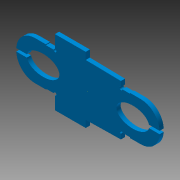
# Autodesk Inventor part: LockZ
Saved by Autodesk Inventor 2014 SP2 (Build 180246200, 246)
## iProperties
Created: 2014-11-24
Part Number: LockZ
Material: Generic
Document SubType Name: Modeling
Designer: JLM
Density: 1 g/cm^3
Appearance: Default
Author: JLM
Autodesk Inventor part; units mm, degrees
ref_plane "YZ Plane" through (0, 0, 0) normal (1, 0, 0) x (0, 1, 0)
ref_plane "XZ Plane" through (0, 0, 0) normal (0, 1, 0) x (-1, 0, 0)
ref_plane "XY Plane" through (0, 0, 0) normal (0, 0, 1) x (1, 0, 0)
sketch "Sketch1" plane through (0, 0, 0) normal (0, 0, 1) x (1, 0, 0)
  line L0 (48.35, 0) -> (48.35, 13.2)
  line L1 (48.35, 13.2) -> (28.35, 13.2)
  line L2 (28.35, 13.2) -> (28.35, 12.7)
  line L3 (28.35, 12.7) -> (22.25, 12.7)
  line L4 (12.2521, 0) -> (48.35, 0)
  line L5 (22.25, 12.7) -> (22.25, 22.25)
  line L6 (22.25, 22.25) -> (0, 22.25)
  line L7 (48.35, 1) -> (41.2045, 1)
  line L8 (48.35, 0) -> (48.35, -13.2)
  line L9 (48.35, -13.2) -> (28.35, -13.2)
  line L10 (28.35, -13.2) -> (28.35, -12.7)
  line L11 (28.35, -12.7) -> (22.25, -12.7)
  line L12 (22.25, -12.7) -> (22.25, -22.25)
  line L13 (22.25, -22.25) -> (0, -22.25)
  line L14 (48.35, -1) -> (41.2045, -1)
  line L15 (0, 22.25) -> (0, -22.25)
  ellipse E0 centre (30.2836, 0) end of major axis (41.3256, 0) minor radius 6.7692 (41.2045, 1) -> (41.2045, -1) ccw
  point P0 (0, 0)
  point P1 (17.8114, 0)
  point P2 (41.275, 1)
  point P3 (41.275, -1)
  dimension "d0" = 13.2
  dimension "d1" = 20
  dimension "d6" = 12.7
  dimension "d7" = 22.25
  dimension "d8" = 22.25
  dimension "d9" = 6.1
  dimension "d17" = 48.35
  dimension "d34" = 1
  constraints: 32 end point, 8 symmetric about line, 7 point on line, 4 perpendicular, 2 parallel, 4 other
  measures "d0" distance of L0.start L0.end
  measures "d1" distance of L0.end L1.end
  measures "d6" distance between parallel lines of L4 L3
  measures "d7" distance between parallel lines of L4 L6
  measures "d8" distance from line of L5 point (0, 0)
  measures "d9" distance of L2.end L3.end
  measures "d17" distance from line of L8 point (0, 0)
  measures "d34" distance between parallel lines of L4 L7
extrude "Extrusion2" add sketch "Sketch1" along normal blind 2.794 contours L7 E0 L14 L8 L9 L10 L11 L12 L13 L15 L6 L5 L3 L2 L1 L0
pattern_circular "Circular Pattern1" count 2 over 360 about axis through (0, 0, -10) along (0, 0, 1) of "Extrusion2"
fillet "Fillet2" radius 12.7 2 edges at (48.35, 13.2, 1.397) (48.35, -13.2, 1.397)
fillet "Fillet3" radius 12.7 2 edges at (-48.35, -13.2, 1.397) (-48.35, 13.2, 1.397)
sketch "Sketch3" plane through (0, 0, 2.794) normal (0, 0, 1) x (1, 0, 0)
  line L0 (22.25, 12.7) -> (22.25, 22.25) projected
  line L1 (22.25, 22.25) -> (-22.25, 22.25) projected
  line L2 (-1.5, 17.5) -> (22.25, 17.0652)
  line L3 (22.25, 22.25) -> (22.25, 17.0652)
  line L4 (0, 0) -> (6.35, 0)
  line L5 (22.25, -12.7) -> (22.25, -22.25)
  line L6 (22.25, -22.25) -> (22.25, -17.0652)
  line L7 (-28.35, 13.2) -> (-35.6598, 13.2) projected
  line L8 (-1.5, 22.25) -> (-1.5, 17.5)
  line L9 (21.8285, 22.25) -> (-1.5, 22.25)
  line L10 (22.25, -12.7) -> (22.25, -22.25)
  line L11 (22.25, -22.25) -> (-22.25, -22.25)
  line L12 (-1.5, -17.5) -> (22.25, -17.0652)
  line L13 (-1.5, -22.25) -> (-1.5, -17.5)
  point P0 (0, 22.25)
  dimension "d32" = 1.5
  dimension "d33" = 17.5
  constraints: 22 end point, 6 point on line, 3 perpendicular, 3 symmetric about line, 1 collinear, 1 midpoint
  measures "d32" distance from line of L4.start L8
  measures "d33" vertical distance of L4.start L2.start
extrude "Extrusion4" cut sketch "Sketch3" against normal up to next
hole "Hole1" at (22.2556, 12.6962, 2.794) direction (0, 0, -1) diameter 2 end through all
mirror "Mirror1" about plane through (0, 0, 0) normal (1, 0, 0) of "Hole1"
mirror "Mirror2" about plane through (0, 0, 0) normal (0, 1, 0) of "Hole1", "Mirror1"
equation "\"d7\" = d8"
body "Solid2"
